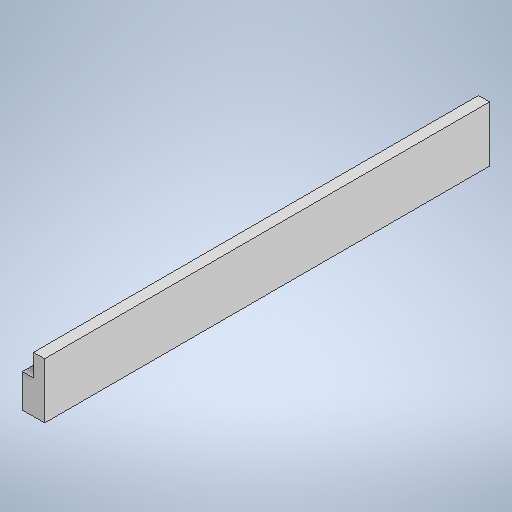
# Autodesk Inventor part: slider_rail
Saved by Autodesk Inventor 2026.1 (Build 301233000, 233)
## iProperties
Created: 2026-05-31
Part Number: slider_rail
Material: Generic
Document SubType Name: Modeling
Designer: chris
Density: 1 g/cm^3
Appearance: Default
Author: chris
Autodesk Inventor part; units mm, degrees
ref_plane "YZ Plane" through (0, 0, 0) normal (1, 0, 0) x (0, 1, 0)
ref_plane "XZ Plane" through (0, 0, 0) normal (0, 1, 0) x (-1, 0, 0)
ref_plane "XY Plane" through (0, 0, 0) normal (0, 0, 1) x (1, 0, 0)
sketch "Sketch1" plane through (0, 0, 0) normal (0, 1, 0) x (-1, 0, 0)
  line L0 (5, 100) -> (-5, 100)
  line L1 (-5, 100) -> (-5, -100)
  line L2 (-5, -100) -> (5, -100)
  line L3 (5, -100) -> (5, 100)
  line L4 (5, 100) -> (-5, -100) construction
  line L5 (-5, 100) -> (5, -100) construction
  point P0 (0, 0)
  dimension "d0" = 10
  dimension "d1" = 200
  constraints: 12 end point, 2 midpoint, 2 parallel, 1 horizontal, 1 perpendicular
  measures "d0" distance of L2.end L1.end
  measures "d1" distance of L1.end L0.end
extrude "Extrusion1" add sketch "Sketch1" along normal blind 15
sketch "Sketch2" plane through (0, 15, 0) normal (0, 1, 0) x (1, 0, 0)
  line L0 (0, -100) -> (5, -100)
  line L1 (5, -100) -> (5, 100)
  line L2 (5, 100) -> (0, 100)
  line L3 (0, 100) -> (0, -100)
  line L4 (5, -100) -> (5, 100) projected
  line L5 (5, 100) -> (-5, 100) projected
  line L6 (-5, -100) -> (5, -100) projected
  point P0 (0, 0)
  dimension "d4" = 5
  constraints: 8 end point, 3 collinear, 2 parallel, 1 horizontal, 1 perpendicular
  measures "d4" distance of L1.end L2.end
extrude "Extrusion2" add sketch "Sketch2" along normal blind 10
body "Solid1"
